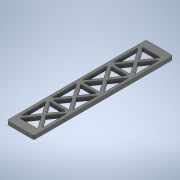
# Autodesk Inventor part: mount_battery_fastener
Saved by Autodesk Inventor 2022.2 (Build 262287000, 287)
## iProperties
Created: 2021-01-30
Part Number: mount_battery_fastener
Material: ABS Plastic
Document SubType Name: Modeling
Designer: User
Density: 1.06 g/cm^3
Appearance: Smooth - Black
Author: User
Autodesk Inventor part; units mm, degrees
ref_plane "YZ Plane" through (0, 0, 0) normal (1, 0, 0) x (0, 1, 0)
ref_plane "XZ Plane" through (0, 0, 0) normal (0, 1, 0) x (-1, 0, 0)
ref_plane "XY Plane" through (0, 0, 0) normal (0, 0, 1) x (1, 0, 0)
sketch "Sketch1" plane through (0, 0, 0) normal (0, 1, 0) x (-1, 0, 0)
  line L0 (-10, 0) -> (-10, 50.8)
  line L1 (-9, 51.8) -> (9, 51.8)
  line L2 (10, 50.8) -> (10, 0)
  line L3 (0, 0) -> (0, 51.8) construction
  arc A0 (-9, 51.8) -> (-10, 50.8) centre (-9, 50.8) ccw
  arc A1 (10, 50.8) -> (9, 51.8) centre (9, 50.8) ccw
  line L4 (10, 0) -> (-10, 0) construction
  line L5 (8, 45.8) -> (-8, 45.8)
  line L6 (8, 45.8) -> (8, 0)
  line L7 (-8, 45.8) -> (-8, 0)
  line L8 (8, 45.8) -> (-8, 22.9) construction
  line L9 (8, 0) -> (-8, 22.9) construction
  line L10 (-8, 0) -> (8, 22.9) construction
  line L11 (-8, 45.8) -> (8, 22.9) construction
  line L12 (-8, 22.9) -> (8, 22.9) construction
  line L13 (8, 1.746) -> (1.2199, 11.45)
  line L14 (1.2199, 11.45) -> (8, 21.154)
  line L15 (8, 24.646) -> (1.2199, 34.35)
  line L16 (1.2199, 34.35) -> (8, 44.054)
  line L17 (-1.2199, 34.35) -> (-8, 24.646)
  line L18 (-1.2199, 34.35) -> (-8, 44.054)
  line L19 (6.0814, 21.9) -> (0, 13.196)
  line L20 (0, 13.196) -> (-6.0814, 21.9)
  line L21 (-6.0814, 21.9) -> (6.0814, 21.9)
  line L22 (6.0814, 23.9) -> (-6.0814, 23.9)
  line L23 (-6.0814, 23.9) -> (0, 32.604)
  line L24 (0, 32.604) -> (6.0814, 23.9)
  line L25 (-1.2199, 11.45) -> (-8, 1.746)
  line L26 (-1.2199, 11.45) -> (-8, 21.154)
  line L27 (0, 36.096) -> (6.7801, 45.8)
  line L28 (0, 36.096) -> (-6.7801, 45.8)
  line L29 (6.0814, 1) -> (-6.0814, 1)
  line L30 (-6.0814, 1) -> (0, 9.704)
  line L31 (6.0814, 1) -> (0, 9.704)
  line L32 (-10, 0) -> (-10, -50.8)
  line L33 (-9, -51.8) -> (9, -51.8)
  line L34 (10, -50.8) -> (10, 0)
  arc A2 (-10, -50.8) -> (-9, -51.8) centre (-9, -50.8) ccw
  arc A3 (9, -51.8) -> (10, -50.8) centre (9, -50.8) ccw
  line L35 (8, -45.8) -> (-8, -45.8)
  line L36 (8, -45.8) -> (8, 0)
  line L37 (-8, -45.8) -> (-8, 0)
  line L38 (8, -45.8) -> (-8, -22.9) construction
  line L39 (8, 0) -> (-8, -22.9) construction
  line L40 (-8, 0) -> (8, -22.9) construction
  line L41 (-8, -45.8) -> (8, -22.9) construction
  line L42 (-8, -22.9) -> (8, -22.9) construction
  line L43 (8, -1.746) -> (1.2199, -11.45)
  line L44 (1.2199, -11.45) -> (8, -21.154)
  line L45 (8, -24.646) -> (1.2199, -34.35)
  line L46 (1.2199, -34.35) -> (8, -44.054)
  line L47 (-1.2199, -34.35) -> (-8, -24.646)
  line L48 (-1.2199, -34.35) -> (-8, -44.054)
  line L49 (6.0814, -21.9) -> (0, -13.196)
  line L50 (0, -13.196) -> (-6.0814, -21.9)
  line L51 (-6.0814, -21.9) -> (6.0814, -21.9)
  line L52 (6.0814, -23.9) -> (-6.0814, -23.9)
  line L53 (-6.0814, -23.9) -> (0, -32.604)
  line L54 (0, -32.604) -> (6.0814, -23.9)
  line L55 (-1.2199, -11.45) -> (-8, -1.746)
  line L56 (-1.2199, -11.45) -> (-8, -21.154)
  line L57 (0, -36.096) -> (6.7801, -45.8)
  line L58 (0, -36.096) -> (-6.7801, -45.8)
  line L59 (6.0814, -1) -> (-6.0814, -1)
  line L60 (-6.0814, -1) -> (0, -9.704)
  line L61 (6.0814, -1) -> (0, -9.704)
  line L62 (-8, 49.8) -> (-6, 49.8)
  line L63 (-6, 49.8) -> (-6, 47.8)
  line L64 (-6, 47.8) -> (-8, 47.8)
  line L65 (-8, 47.8) -> (-8, 49.8)
  line L66 (-8, 47.8) -> (-8, 45.8)
  line L67 (-8, 49.8) -> (-8, 51.8)
  line L68 (-8, -49.8) -> (-6, -49.8)
  line L69 (-6, -49.8) -> (-6, -47.8)
  line L70 (-6, -47.8) -> (-8, -47.8)
  line L71 (-8, -47.8) -> (-8, -49.8)
  point P0 (-10, 51.8)
  point P1 (10, 51.8)
  point P2 (0, 0)
  point P3 (-10, -51.8)
  point P4 (10, -51.8)
  point P5 (0, -51.8)
  dimension "d6" = 20
  dimension "d11" = 1
  dimension "d21" = 2
  dimension "d22" = 2
  dimension "d23" = 2
  dimension "d25" = 2
  dimension "d26" = 2
  dimension "d28" = 2
  dimension "d29" = 2
  dimension "d30" = 2
  dimension "d31" = 2
  dimension "d32" = 2
  dimension "d33" = 2
  dimension "d38" = 2
  dimension "d39" = 2
  dimension "d40" = 2
  dimension "d41" = 2
  dimension "d42" = 2
  dimension "d43" = 2
  dimension "d47" = 2
  dimension "d48" = 2
  dimension "d53" = 50.8
  dimension "d54" = 6
  constraints: 144 end point, 41 symmetric about line, 32 point on line, 19 parallel, 8 point on circle, 7 midpoint, 6 perpendicular, 5 horizontal, 4 centre point, 4 horizontal alignment, 4 tangent, 2 equal length, 2 vertical, 2 vertical alignment, 1 equal radius, 3 other
  measures "d6" distance of point (-10, 51.8) point (10, 51.8)
  measures "d11" radius of A0
  measures "d21" distance between parallel lines of L0 L7
  measures "d22" distance between parallel lines of L2 L6
  measures "d23" diameter of L13 L9
  measures "d25" diameter of L14 L10
  measures "d26" diameter of L19 L10
  measures "d28" diameter of L25 L10
  measures "d29" diameter of L21 L12
  measures "d30" diameter of L22 L12
  measures "d31" diameter of L24 L11
  measures "d32" diameter of L15 L11
  measures "d33" diameter of L16 L8
  measures "d38" diameter of L18 L11
  measures "d39" diameter of L17 L8
  measures "d40" diameter of L28 L11
  measures "d41" diameter of L26 L9
  measures "d42" diameter of L29 L4
  measures "d43" diameter of L31 L9
  measures "d47" distance of L64.end L62.start
  measures "d48" distance of L62.start L62.end
  measures "d53" distance of L0.start L32.end
  measures "d54" distance between parallel lines of L1 L5
extrude "Extrusion2" add sketch "Sketch1" along normal blind 2.7 contours L0 A0 L1 A1 L2 L34 A3 L33 A2 L32 | L6 L16 L15 L14 L13 L36 L43 L44 L45 L46 L35 L57 L58 L37 L48 L47 L56 L55 L7 L25 L26 L17 L18 L5 L28 L27 | L62 L63 L64 L65 | L71 L70 L69 L68
fillet "Fillet1" radius 0.4 47 edges at (-8, 1.35, 44.054) (-8, 1.35, 24.646) (-1.2199, 1.35, 34.35) (-6.7801, 1.35, 45.8) (0, 1.35, 36.096) (6.7801, 1.35, 45.8) (8, 1.35, 44.054) (1.2199, 1.35, 34.35) (0, 1.35, 32.604) (6.0814, 1.35, 23.9) (8, 1.35, 24.646) (6.0814, 1.35, 21.9) (-6.0814, 1.35, 21.9) (-8, 1.35, 21.154) (0, 1.35, 13.196) (-1.2199, 1.35, 11.45) (6.0814, 1.35, 1) (-6.0814, 1.35, 1) (-8, 1.35, 1.746) (0, 1.35, 9.704) (1.2199, 1.35, 11.45) (8, 1.35, 1.746) (8, 1.35, 21.154) (-6.0814, 1.35, -1) (0, 1.35, -9.704) (6.0814, 1.35, -1) (8, 1.35, -1.746) (1.2199, 1.35, -11.45) (-1.2199, 1.35, -11.45) (-8, 1.35, -1.746) (-8, 1.35, -21.154) (-6.0814, 1.35, -21.9) (6.0814, 1.35, -21.9) (0, 1.35, -13.196) (8, 1.35, -21.154) (-6.0814, 1.35, -23.9) (0, 1.35, -32.604) (6.0814, 1.35, -23.9) (8, 1.35, -24.646) (1.2199, 1.35, -34.35) (8, 1.35, -44.054) (6.7801, 1.35, -45.8) (-6.7801, 1.35, -45.8) (0, 1.35, -36.096) (-8, 1.35, -44.054) (-8, 1.35, -24.646) (-1.2199, 1.35, -34.35)
equation "\"d21\" = link_width"
equation "\"d22\" = link_width"
equation "\"d23\" = link_width"
equation "\"d25\" = link_width"
equation "\"d26\" = link_width"
equation "\"d28\" = link_width"
equation "\"d29\" = link_width"
equation "\"d30\" = link_width"
equation "\"d31\" = link_width"
equation "\"d32\" = link_width"
equation "\"d33\" = link_width"
equation "\"d38\" = link_width"
equation "\"d39\" = link_width"
equation "\"d40\" = link_width"
equation "\"d41\" = link_width"
equation "\"d42\" = link_width"
equation "\"d43\" = link_width"
equation "\"link_width\" = 2"
body "Solid2"
